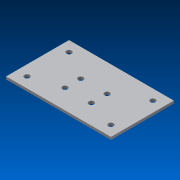
# Autodesk Inventor part: CylinderPlate
Saved by Autodesk Inventor 2013 (Build 170138000, 138)
## iProperties
Created: 2013-07-19
Part Number: CylinderPlate
Material: Aluminum 6061
Document SubType Name: Modeling
Designer: robotics
Density: 1 g/cm^3
Author: robotics
Autodesk Inventor part; units mm, degrees
ref_plane "YZ Plane" through (0, 0, 0) normal (1, 0, 0) x (0, 1, 0)
ref_plane "XZ Plane" through (0, 0, 0) normal (0, 1, 0) x (-1, 0, 0)
ref_plane "XY Plane" through (0, 0, 0) normal (0, 0, 1) x (1, 0, 0)
sketch "Sketch1" plane through (0, 0, 0) normal (0, 1, 0) x (-1, 0, 0)
  line L0 (0, 0) -> (127, 0)
  line L1 (127, 0) -> (127, 76.2)
  line L2 (127, 76.2) -> (0, 76.2)
  line L3 (0, 76.2) -> (0, 0)
  dimension "d0" = 76.2
  dimension "d2" = 127
  constraints: 8 end point, 2 parallel, 1 horizontal, 1 perpendicular
  measures "d0" distance of L0.end L1.end
  measures "d2" distance of L1.end L2.end
extrude "Extrusion1" add sketch "Sketch1" along normal blind 3.175
sketch "Sketch2" plane through (0, 3.175, 0) normal (0, 1, 0) x (1, 0, 0)
  line L0 (0, 0) -> (-127, 0) projected
  line L1 (-127, 0) -> (-127, -76.2) projected
  line L2 (-127, -76.2) -> (0, -76.2) projected
  line L3 (0, -76.2) -> (0, 0) projected
  point P0 (-114.3, -12.7)
  point P1 (-114.3, -63.5)
  point P2 (-12.7, -63.5)
  point P3 (-12.7, -12.7)
  dimension "d5" = 12.7
  dimension "d6" = 12.7
  dimension "d7" = 12.7
  dimension "d8" = 12.7
  dimension "d9" = 12.7
  dimension "d10" = 12.7
  dimension "d11" = 12.7
  dimension "d12" = 12.7
  dimension "d13" = 50.8
  dimension "d14" = 101.6
  dimension "d15" = 50.8
  measures "d5" distance from line of point (-114.3, -12.7) L1
  measures "d6" distance from line of point (-114.3, -12.7) L0
  measures "d7" distance from line of point (-114.3, -63.5) L2
  measures "d8" distance from line of L1 point (-114.3, -63.5)
  measures "d9" distance from line of point (-12.7, -12.7) L3
  measures "d10" distance from line of point (-12.7, -12.7) L0
  measures "d11" distance from line of L3 point (-12.7, -63.5)
  measures "d12" distance from line of L2 point (-12.7, -63.5)
  measures "d13" distance of point (-12.7, -63.5) point (-12.7, -12.7)
  measures "d14" distance of point (-114.3, -12.7) point (-12.7, -12.7)
  measures "d15" distance of point (-114.3, -12.7) point (-114.3, -63.5)
hole "Hole1" at (-114.3, 3.175, 12.7) at (-114.3, 3.175, 63.5) at (-12.7, 3.175, 63.5) at (-12.7, 3.175, 12.7) direction (0, -1, 0) diameter 6.35 end through all
sketch "Sketch3" plane through (0, 3.175, 0) normal (0, 1, 0) x (1, 0, 0)
  line L0 (-127, 0) -> (-127, -76.2) projected
  line L1 (-127, -76.2) -> (0, -76.2) projected
  line L2 (0, -76.2) -> (0, 0) projected
  point P0 (-79.4512, -52.3748)
  point P1 (-47.5488, -52.3748)
  point P2 (-79.4512, -33.3248)
  point P3 (-47.5488, -33.3248)
  dimension "d23" = 47.5488
  dimension "d24" = 47.5488
  dimension "d25" = 47.5488
  dimension "d26" = 47.5488
  dimension "d27" = 19.05
  dimension "d28" = 19.05
  dimension "d29" = 23.8252
  dimension "d30" = 23.8252
  measures "d23" distance from line of L0 point (-79.451, -33.325)
  measures "d24" distance from line of point (-79.451, -52.375) L0
  measures "d25" distance from line of L2 point (-47.549, -33.325)
  measures "d26" distance from line of L2 point (-47.549, -52.375)
  measures "d27" distance of point (-79.451, -52.375) point (-79.451, -33.325)
  measures "d28" distance of point (-47.549, -52.375) point (-47.549, -33.325)
  measures "d29" distance from line of L1 point (-79.451, -52.375)
  measures "d30" distance from line of L1 point (-47.549, -52.375)
hole "Hole2" at (-79.4512, 3.175, 52.3748) at (-47.5488, 3.175, 52.3748) at (-79.4512, 3.175, 33.3248) at (-47.5488, 3.175, 33.3248) direction (0, -1, 0) diameter 6.35 end through all
body "Solid1"
